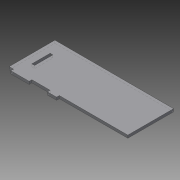
# Autodesk Inventor part: Frount plate
Saved by Autodesk Inventor 2015 (Build 190159000, 159)
## iProperties
Created: 2014-08-15
Part Number: Frount plate
Material: Generic
Document SubType Name: Modeling
Designer: karl
Density: 1 g/cm^3
Appearance: Default
Author: karl
Autodesk Inventor part; units mm, degrees
ref_plane "YZ Plane" through (0, 0, 0) normal (1, 0, 0) x (0, 1, 0)
ref_plane "XZ Plane" through (0, 0, 0) normal (0, 1, 0) x (-1, 0, 0)
ref_plane "XY Plane" through (0, 0, 0) normal (0, 0, 1) x (1, 0, 0)
sketch "Sketch1" plane through (0, 0, 0) normal (0, 0, 1) x (1, 0, 0)
  circle A0 centre (0, 0) radius 85 construction
  line L0 (-64.8074, 55) -> (64.8074, 55) construction
  line L1 (64.8074, -25) -> (-64.8074, -25)
  line L2 (-64.8074, -25) -> (-64.8074, 25)
  line L3 (-64.8074, 25) -> (64.8074, 25)
  line L4 (64.8074, 25) -> (64.8074, -25)
  line L5 (64.8074, -25) -> (-64.8074, 25) construction
  line L6 (-64.8074, -25) -> (64.8074, 25) construction
  dimension "d0" = 170
  dimension "d1" = 55
  dimension "d2" = 129.6148
  dimension "d3" = 50
  constraints: 14 end point, 3 parallel, 2 horizontal, 2 midpoint, 2 point on circle, 1 centre point, 1 coincident, 1 perpendicular
  measures "d0" diameter of A0
  measures "d1" distance from line of L0 point (0, 0)
  measures "d2" distance of L0.start L0.end
  measures "d3" distance of L1.end L2.end
extrude "Extrusion1" add sketch "Sketch1" along normal blind 3
sketch "Sketch2" plane through (0, 0, 3) normal (0, 0, 1) x (1, 0, 0)
  line L0 (-64.8074, -25) -> (64.8074, -25) projected
  line L1 (-40, -25) -> (-60, -25)
  line L2 (-60, -25) -> (-60, -28)
  line L3 (-60, -28) -> (-40, -28)
  line L4 (-40, -28) -> (-40, -25)
  line L5 (-20, -25) -> (-10, -25)
  line L6 (-10, -25) -> (-10, -28)
  line L7 (-10, -28) -> (-20, -28)
  line L8 (-20, -28) -> (-20, -25)
  point P0 (0, 0)
  dimension "d6" = 20
  dimension "d7" = 3
  dimension "d8" = 10
  dimension "d9" = 3
  dimension "d10" = 10
  dimension "d11" = 20
  constraints: 16 end point, 4 parallel, 2 horizontal, 2 perpendicular, 2 point on line
  measures "d6" distance of L3.end L2.end
  measures "d7" distance of L2.end L1.end
  measures "d8" distance of L6.end L7.end
  measures "d9" distance of L5.end L6.end
  measures "d10" distance from line of point (0, 0) L6
  measures "d11" distance between parallel lines of L8 L4
extrude "Extrusion2" add sketch "Sketch2" against normal blind 3
sketch "Sketch3" plane through (0, 0, 3) normal (0, 0, 1) x (1, 0, 0)
  line L0 (-60, 10) -> (-57, 10)
  line L1 (-57, 10) -> (-57, -10)
  line L2 (-57, -10) -> (-60, -10)
  line L3 (-60, -10) -> (-60, 10)
  point P0 (0, 0)
  point P1 (-60, 0)
  dimension "d14" = 3
  dimension "d15" = 20
  dimension "d16" = 57
  constraints: 8 end point, 2 parallel, 1 horizontal, 1 horizontal alignment, 1 midpoint, 1 perpendicular
  measures "d14" distance of L1.end L2.end
  measures "d15" distance of L0.end L1.end
  measures "d16" distance from line of point (0, 0) L1
extrude "Extrusion3" cut sketch "Sketch3" against normal blind 3
mirror "Mirror1" about plane through (0, 0, 0) normal (1, 0, 0) of "Extrusion2", "Extrusion3"
body "Solid1"
